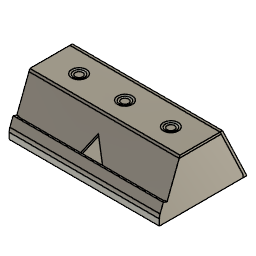
E-paper_v3 (Autodesk Fusion 360 design; units mm, degrees)
Autodesk Fusion 360 part; units mm, degrees
sketch "Sketch1" plane through (0, 0, 0) normal (1, 0, 0) x (0, 1, 0)
  line L0 (0, 0) -> (-90, 0)
  line L1 (-90, 0) -> (-54.1632, 93.358)
  line L2 (-90, 0) -> (10, 0) construction
  line L3 (0, -3.5) -> (-95.0925, -3.5)
  line L4 (-95.0925, -3.5) -> (-57.4307, 94.6123)
  line L5 (-58.8311, 95.1499) -> (-96.6992, -3.5)
  line L6 (-96.6992, -3.5) -> (-95.0925, -3.5)
  line L7 (-93.749, 0) -> (-95.3557, 0)
  line L8 (-96.6992, -3.5) -> (-100.1992, -3.5)
  line L9 (-100.1992, -3.5) -> (-62.3311, 95.1499)
  line L10 (-95.3557, 0) -> (-98.8557, 0)
  line L11 (-98.8557, 0) -> (-95.4512, 8.869)
  line L12 (-95.4512, 8.869) -> (-92.4007, 7.698)
  line L13 (-57.4307, 94.6123) -> (-54.1632, 93.358)
  line L14 (0, -3.5) -> (0, 0)
  line L15 (-92.4007, 7.698) -> (-91.0004, 7.1605)
  line L16 (-54.1632, 93.358) -> (0, 0)
  line L17 (-100.1992, -3.5) -> (0, -3.5) construction
  line L18 (0, -3.5) -> (0, -13.5)
  line L19 (0, -13.5) -> (-100.1992, -13.5)
  line L20 (-100.1992, -13.5) -> (-100.1992, -3.5)
  line L21 (0, -13.5) -> (0, -10)
  line L22 (0, -10) -> (-90, -10)
  line L23 (-90, -10) -> (-90, 0)
  dimension "d1" = 90
  dimension "d3" = 69
  dimension "d4" = 100
  dimension "d5" = -3.5
  dimension "d6" = 1.5
  dimension "d7" = 3.5
  dimension "d8" = 9.5
  dimension "d13" = 10
  dimension "d14" = 3.5
  constraint coincident L0.start L14.end
  constraint horizontal L0
  constraint horizontal L2
  constraint parallel L3 L6
  constraint coincident L4 L7.start
  constraint coincident L5 L7.end
  constraint parallel L6 L7
  constraint parallel L6 L8
  constraint parallel L5 L9
  constraint coincident L9 L10.end
  constraint parallel L7 L10
  constraint parallel L9 L11
  constraint coincident L5 L12.end
  constraint perpendicular L5 L12
  constraint perpendicular L1 L13
  constraint perpendicular L0 L14
  constraint coincident L4 L15.end
  constraint perpendicular L4 L15
  constraint horizontal L17
  constraint vertical L18
  constraint horizontal L19
  constraint vertical L20
  constraint perpendicular L19 L21
  constraint perpendicular L21 L22
  constraint perpendicular L17 L23
  measures "d1" distance of L0.start L0.end
  measures "d3" angle of L1 L2
  measures "d4" distance of L0.end L1.end
  measures "d6" distance of L4.end L5.start
  measures "d7" distance of L5.end L8.end
  measures "d8" distance of L10.end L11.end
  measures "d13" distance of L8.end L19.end
  measures "d14" distance of L18.end L21.end
extrude "Extrude1" add sketch "Sketch1" along normal blind 3 makes body 1
extrude "Extrude2" add sketch "Sketch1" against normal blind 174 contours L1 L3 L4 L13 L23 | L3 L6 L8 L18 L19 L20 L21 L22 L23 | L4 L5 L6 L7 | L5 L8 L9 L10 | L5 L9 L10 L11 L12 bodies 1
extrude "Extrude3" add sketch "Sketch1" against normal blind 3 from surface at -174 bodies 1
ref_plane "WorkPlane1" through (-87, -50.0996, 40.5562) normal (-1, 0, 0) x (0, 0, 1)
sketch "Sketch2" plane through (-87, 0, 0) normal (-1, 0, 0) x (0, -1, 0)
  arc A0 (90, -3.5) -> (95.35, 0) centre (90.3987, 1.7294) ccw
  line L0 (95.35, 0) -> (89.5, 0)
  line L1 (89.5, 0) -> (89.5, -3.5)
  line L2 (89.5, -3.5) -> (90, -3.5)
  constraint horizontal L0
  constraint perpendicular L0 L1
extrude "Extrude4" cut sketch "Sketch2" along normal mid plane 34 bodies 1
sketch "Sketch3" plane through (0, -81.709, 31.3652) normal (0, -0.93358, 0.358368) x (1, 0, 0)
  line L0 (0, -25.9267) -> (3, -25.9267)
  line L1 (3, -25.9267) -> (3, 67.7469)
  line L2 (3, 67.7469) -> (-177, 67.7469)
  line L3 (-177, 67.7469) -> (-177, -25.9267)
  line L4 (-177, -25.9267) -> (-174, -25.9267)
  line L5 (-174, -25.9267) -> (-174, -33.5966)
  line L6 (-174, -33.5966) -> (-104, -33.5966)
  line L7 (-104, -33.5966) -> (-70, -33.5966)
  line L8 (-70, -33.5966) -> (0, -33.5966)
  line L9 (0, -33.5966) -> (0, -25.9267)
  line L10 (-104, -33.5966) -> (-87.5, -3)
  line L11 (-87.5, -3) -> (-70, -33.5966)
  line L12 (-104, -33.5966) -> (-70, -33.5966)
  constraint coincident L6.end L7.start
  constraint coincident L7.end L8.start
extrude "Extrude5" cut sketch "Sketch3" against normal blind 5 contours L7 L10 L11 L12 bodies 1
sketch "Sketch4" plane through (0, -90, 0) normal (0, 1, 0) x (-1, 0, 0)
  line L0 (104, 0) -> (104, -3.5)
  line L1 (104, -3.5) -> (70, -3.5)
  line L2 (70, -3.5) -> (70, 0)
  line L3 (70, 0) -> (0, 0)
  line L4 (0, 0) -> (0, -10)
  line L5 (0, -10) -> (174, -10)
  line L6 (174, -10) -> (174, 0)
  line L7 (174, 0) -> (104, 0)
  line L8 (12.6874, -4.866) -> (9.8668, -2.0298)
  line L9 (9.8668, -2.0298) -> (7.0306, -4.8504)
  line L10 (7.0306, -4.8504) -> (9.8511, -7.6866)
  line L11 (9.8511, -7.6866) -> (12.6874, -4.866)
  line L12 (40.6511, -7.6866) -> (43.4874, -4.866)
  line L13 (37.8306, -4.8504) -> (40.6511, -7.6866)
  line L14 (40.6668, -2.0298) -> (37.8306, -4.8504)
  line L15 (43.4874, -4.866) -> (40.6668, -2.0298)
  line L16 (71.4511, -7.6866) -> (74.2874, -4.866)
  line L17 (68.6306, -4.8504) -> (71.4511, -7.6866)
  line L18 (71.4668, -2.0298) -> (68.6306, -4.8504)
  line L19 (74.2874, -4.866) -> (71.4668, -2.0298)
  line L20 (102.2511, -7.6866) -> (105.0874, -4.866)
  line L21 (99.4306, -4.8504) -> (102.2511, -7.6866)
  line L22 (102.2668, -2.0298) -> (99.4306, -4.8504)
  line L23 (105.0874, -4.866) -> (102.2668, -2.0298)
  line L24 (133.0511, -7.6866) -> (135.8874, -4.866)
  line L25 (130.2306, -4.8504) -> (133.0511, -7.6866)
  line L26 (133.0668, -2.0298) -> (130.2306, -4.8504)
  line L27 (135.8874, -4.866) -> (133.0668, -2.0298)
  line L28 (163.8511, -7.6866) -> (166.6874, -4.866)
  line L29 (161.0306, -4.8504) -> (163.8511, -7.6866)
  line L30 (163.8668, -2.0298) -> (161.0306, -4.8504)
  line L31 (166.6874, -4.866) -> (163.8668, -2.0298)
  point P0 (9.859, -4.8582)
  point P1 (40.659, -4.8582)
  point P2 (71.459, -4.8582)
  point P3 (102.259, -4.8582)
  point P4 (133.059, -4.8582)
  point P5 (163.859, -4.8582)
  dimension "d22" = 2
  dimension "d25" = 154
  dimension "d26" = 0
  measures "d22" distance of P0 L11
sketch "Sketch5" plane through (0, -90, 0) normal (0, 1, 0) x (-1, 0, 0)
extrude "Extrude6" cut sketch "Sketch4" against normal blind 8.8 contours L1 L20 L21 L22 L23 | L1 L22 L23 | L1 L2 L16 L17 L18 L19 | L1 L2 L18 L19 | L8 L9 L10 L11 | L12 L13 L14 L15 | L24 L25 L26 L27 | L28 L29 L30 L31 bodies 1
sketch "Sketch6" plane through (3, 0, 0) normal (1, 0, 0) x (0, 1, 0)
  line L0 (-100.1992, -13.5) -> (0, -13.5)
  line L1 (0, -13.5) -> (0, 0)
  line L2 (0, 0) -> (-54.1632, 93.358)
  line L3 (-54.1632, 93.358) -> (-57.4307, 94.6123)
  line L4 (-57.4307, 94.6123) -> (-91.0004, 7.1605)
  line L5 (-91.0004, 7.1605) -> (-95.4512, 8.869)
  line L6 (-95.4512, 8.869) -> (-100.1992, -3.5)
  line L7 (-100.1992, -3.5) -> (-100.1992, -13.5)
  line L8 (-100, 45) -> (0, 45)
  line L9 (0, 45) -> (0, 100)
  line L10 (0, 100) -> (-100, 100)
  line L11 (-100, 100) -> (-100, 45)
  constraint horizontal L8
  constraint vertical L9
  constraint horizontal L10
  constraint vertical L11
extrude "Extrude7" cut sketch "Sketch6" against normal blind 200 contours L2 L3 L4 L8 bodies 1
fillet "Fillet1" radius 13 1 edges at (-87, -100.1992, -3.5) on bodies 1
sketch "Sketch7" plane through (-177, 0, 0) normal (-1, 0, 0) x (0, -1, 0)
  arc A0 (100.1992, -5.9094) -> (99.3358, -1.2506) centre (87.1992, -5.9094) ccw
  line L0 (99.3358, -1.2506) -> (95.4512, 8.869)
  line L1 (95.4512, 8.869) -> (91.0004, 7.1605)
  line L2 (91.0004, 7.1605) -> (76.4751, 45)
  line L3 (76.4751, 45) -> (26.1075, 45)
  line L4 (26.1075, 45) -> (0, 0)
  line L5 (0, 0) -> (0, -13.5)
  line L6 (0, -13.5) -> (100.1992, -13.5)
  line L7 (100.1992, -13.5) -> (100.1992, -5.9094)
  line L8 (0, -10) -> (26.1075, 45)
  line L9 (-5, 45) -> (26.1075, 45)
  line L10 (-5, 45) -> (0, -10)
  constraint coincident L5 L8.start
  constraint coincident L3.end L4.start
  constraint parallel L3 L9
extrude "Extrude8" cut sketch "Sketch7" against normal blind 225 contours L4 L5 L8 bodies 1
sketch "Sketch8" plane through (0, 0, -13.5) normal (0, 0, -1) x (1, 0, 0)
  line L0 (-177, 0) -> (3, 0)
  line L1 (3, 0) -> (3, 100.1992)
  line L2 (3, 100.1992) -> (-177, 100.1992)
  line L3 (-177, 100.1992) -> (-177, 0)
  line L4 (-25, 60) -> (-28.8404, 50)
  line L5 (-28.8404, 50) -> (-30.266, 50)
  line L6 (-30.266, 50) -> (-34.3588, 60)
  line L7 (-34.3588, 60) -> (-32.8513, 60)
  line L8 (-32.8513, 60) -> (-31.6849, 56.9714)
  line L9 (-31.6849, 56.9714) -> (-27.5034, 56.9714)
  line L10 (-27.5034, 56.9714) -> (-26.4052, 60)
  line L11 (-26.4052, 60) -> (-25, 60)
  line L12 (-27.8854, 55.8936) -> (-31.2756, 55.8936)
  line L13 (-31.2756, 55.8936) -> (-30.2319, 53.1241)
  spline S0 degree 2 poles (-30.2319, 53.1241) (-29.7544, 51.8622) (-29.5225, 51.0505) knots 0 0 0 1 1 1
  spline S1 degree 2 poles (-29.5225, 51.0505) (-29.3315, 52.0123) (-28.9836, 52.9604) knots 0 0 0 1 1 1
  line L14 (-28.9836, 52.9604) -> (-27.8854, 55.8936)
  line L15 (-35.2319, 60) -> (-35.2319, 50)
  line L16 (-35.2319, 50) -> (-36.4598, 50)
  line L17 (-36.4598, 50) -> (-36.4598, 60)
  line L18 (-36.4598, 60) -> (-35.2319, 60)
  line L19 (-43.322, 57.6671) -> (-44.5907, 57.824)
  spline S2 degree 2 poles (-44.5907, 57.824) (-44.2906, 58.9359) (-43.4789, 59.5498) knots 0 0 0 1 1 1
  spline S3 degree 2 poles (-43.4789, 59.5498) (-42.6671, 60.1637) (-41.4052, 60.1637) knots 0 0 0 1 1 1
  spline S4 degree 2 poles (-41.4052, 60.1637) (-39.8158, 60.1637) (-38.8847, 59.1849) knots 0 0 0 1 1 1
  spline S5 degree 2 poles (-38.8847, 59.1849) (-37.9536, 58.206) (-37.9536, 56.4393) knots 0 0 0 1 1 1
  spline S6 degree 2 poles (-37.9536, 56.4393) (-37.9536, 54.6112) (-38.895, 53.6016) knots 0 0 0 1 1 1
  spline S7 degree 2 poles (-38.895, 53.6016) (-39.8363, 52.5921) (-41.337, 52.5921) knots 0 0 0 1 1 1
  spline S8 degree 2 poles (-41.337, 52.5921) (-42.7899, 52.5921) (-43.7108, 53.5812) knots 0 0 0 1 1 1
  spline S9 degree 2 poles (-43.7108, 53.5812) (-44.6317, 54.5703) (-44.6317, 56.3643) knots 0 0 0 1 1 1
  spline S10 degree 2 poles (-44.6317, 56.3643) (-44.6317, 56.4734) (-44.6248, 56.6917) knots 0 0 0 1 1 1
  line L20 (-44.6248, 56.6917) -> (-39.2224, 56.6917)
  spline S11 degree 2 poles (-39.2224, 56.6917) (-39.2906, 57.8854) (-39.8977, 58.5198) knots 0 0 0 1 1 1
  spline S12 degree 2 poles (-39.8977, 58.5198) (-40.5048, 59.1542) (-41.412, 59.1542) knots 0 0 0 1 1 1
  spline S13 degree 2 poles (-41.412, 59.1542) (-42.0873, 59.1542) (-42.5648, 58.7995) knots 0 0 0 1 1 1
  spline S14 degree 2 poles (-42.5648, 58.7995) (-43.0423, 58.4447) (-43.322, 57.6671) knots 0 0 0 1 1 1
  line L21 (-39.2906, 55.6821) -> (-43.3356, 55.6821)
  spline S15 degree 2 poles (-43.3356, 55.6821) (-43.2538, 54.7681) (-42.8718, 54.3111) knots 0 0 0 1 1 1
  spline S16 degree 2 poles (-42.8718, 54.3111) (-42.2851, 53.6016) (-41.3506, 53.6016) knots 0 0 0 1 1 1
  spline S17 degree 2 poles (-41.3506, 53.6016) (-40.5048, 53.6016) (-39.9284, 54.1678) knots 0 0 0 1 1 1
  spline S18 degree 2 poles (-39.9284, 54.1678) (-39.352, 54.734) (-39.2906, 55.6821) knots 0 0 0 1 1 1
  line L22 (-54.8499, 56.0778) -> (-54.8499, 54.9045)
  line L23 (-54.8499, 54.9045) -> (-59.0859, 54.8977)
  line L24 (-59.0859, 54.8977) -> (-59.0859, 58.6085)
  spline S19 degree 2 poles (-59.0859, 58.6085) (-58.1105, 59.3861) (-57.0737, 59.7783) knots 0 0 0 1 1 1
  spline S20 degree 2 poles (-57.0737, 59.7783) (-56.0368, 60.1705) (-54.9454, 60.1705) knots 0 0 0 1 1 1
  spline S21 degree 2 poles (-54.9454, 60.1705) (-53.472, 60.1705) (-52.2681, 59.5396) knots 0 0 0 1 1 1
  spline S22 degree 2 poles (-52.2681, 59.5396) (-51.0641, 58.9086) (-50.4502, 57.7149) knots 0 0 0 1 1 1
  spline S23 degree 2 poles (-50.4502, 57.7149) (-49.8363, 56.5211) (-49.8363, 55.0478) knots 0 0 0 1 1 1
  spline S24 degree 2 poles (-49.8363, 55.0478) (-49.8363, 53.588) (-50.4468, 52.3226) knots 0 0 0 1 1 1
  spline S25 degree 2 poles (-50.4468, 52.3226) (-51.0573, 51.0573) (-52.2033, 50.4434) knots 0 0 0 1 1 1
  spline S26 degree 2 poles (-52.2033, 50.4434) (-53.3493, 49.8295) (-54.8431, 49.8295) knots 0 0 0 1 1 1
  spline S27 degree 2 poles (-54.8431, 49.8295) (-55.9277, 49.8295) (-56.8042, 50.1808) knots 0 0 0 1 1 1
  spline S28 degree 2 poles (-56.8042, 50.1808) (-57.6808, 50.5321) (-58.1787, 51.1596) knots 0 0 0 1 1 1
  spline S29 degree 2 poles (-58.1787, 51.1596) (-58.6767, 51.7872) (-58.9359, 52.7967) knots 0 0 0 1 1 1
  line L25 (-58.9359, 52.7967) -> (-57.7422, 53.1241)
  spline S30 degree 2 poles (-57.7422, 53.1241) (-57.5171, 52.3602) (-57.1828, 51.9236) knots 0 0 0 1 1 1
  spline S31 degree 2 poles (-57.1828, 51.9236) (-56.8486, 51.487) (-56.2278, 51.2244) knots 0 0 0 1 1 1
  spline S32 degree 2 poles (-56.2278, 51.2244) (-55.6071, 50.9618) (-54.8499, 50.9618) knots 0 0 0 1 1 1
  spline S33 degree 2 poles (-54.8499, 50.9618) (-53.9427, 50.9618) (-53.281, 51.2381) knots 0 0 0 1 1 1
  spline S34 degree 2 poles (-53.281, 51.2381) (-52.6194, 51.5143) (-52.2135, 51.9645) knots 0 0 0 1 1 1
  spline S35 degree 2 poles (-52.2135, 51.9645) (-51.8076, 52.4147) (-51.5825, 52.9536) knots 0 0 0 1 1 1
  spline S36 degree 2 poles (-51.5825, 52.9536) (-51.2005, 53.8813) (-51.2005, 54.9659) knots 0 0 0 1 1 1
  spline S37 degree 2 poles (-51.2005, 54.9659) (-51.2005, 56.3029) (-51.661, 57.2033) knots 0 0 0 1 1 1
  spline S38 degree 2 poles (-51.661, 57.2033) (-52.1214, 58.1037) (-53.0014, 58.5402) knots 0 0 0 1 1 1
  spline S39 degree 2 poles (-53.0014, 58.5402) (-53.8813, 58.9768) (-54.8704, 58.9768) knots 0 0 0 1 1 1
  spline S40 degree 2 poles (-54.8704, 58.9768) (-55.7299, 58.9768) (-56.5484, 58.646) knots 0 0 0 1 1 1
  spline S41 degree 2 poles (-56.5484, 58.646) (-57.367, 58.3151) (-57.7899, 57.94) knots 0 0 0 1 1 1
  line L26 (-57.7899, 57.94) -> (-57.7899, 56.0778)
  line L27 (-57.7899, 56.0778) -> (-54.8499, 56.0778)
  spline S42 degree 2 poles (-32.94, 74.4952) (-32.4966, 75.0068) (-31.9475, 75.3172) knots 0 0 0 1 1 1
  spline S43 degree 2 poles (-31.9475, 75.3172) (-31.3984, 75.6276) (-30.8458, 75.6276) knots 0 0 0 1 1 1
  spline S44 degree 2 poles (-30.8458, 75.6276) (-30.2387, 75.6276) (-29.6658, 75.2729) knots 0 0 0 1 1 1
  spline S45 degree 2 poles (-29.6658, 75.2729) (-29.0928, 74.9181) (-28.7347, 74.1814) knots 0 0 0 1 1 1
  spline S46 degree 2 poles (-28.7347, 74.1814) (-28.3765, 73.4447) (-28.3765, 72.5648) knots 0 0 0 1 1 1
  spline S47 degree 2 poles (-28.3765, 72.5648) (-28.3765, 71.4802) (-28.9325, 70.3922) knots 0 0 0 1 1 1
  spline S48 degree 2 poles (-28.9325, 70.3922) (-29.4884, 69.3042) (-30.3138, 68.7585) knots 0 0 0 1 1 1
  spline S49 degree 2 poles (-30.3138, 68.7585) (-31.1392, 68.2128) (-31.9168, 68.2128) knots 0 0 0 1 1 1
  spline S50 degree 2 poles (-31.9168, 68.2128) (-32.5102, 68.2128) (-33.0491, 68.5232) knots 0 0 0 1 1 1
  spline S51 degree 2 poles (-33.0491, 68.5232) (-33.588, 68.8336) (-33.9768, 69.4679) knots 0 0 0 1 1 1
  line L28 (-33.9768, 69.4679) -> (-34.2087, 68.4106)
  line L29 (-34.2087, 68.4106) -> (-35.4297, 68.4106)
  line L30 (-35.4297, 68.4106) -> (-34.4475, 72.9877)
  spline S52 degree 2 poles (-34.4475, 72.9877) (-34.2428, 73.9427) (-34.2428, 74.045) knots 0 0 0 1 1 1
  spline S53 degree 2 poles (-34.2428, 74.045) (-34.2428, 74.2292) (-34.3827, 74.3622) knots 0 0 0 1 1 1
  spline S54 degree 2 poles (-34.3827, 74.3622) (-34.5225, 74.4952) (-34.7203, 74.4952) knots 0 0 0 1 1 1
  spline S55 degree 2 poles (-34.7203, 74.4952) (-35.0819, 74.4952) (-35.6685, 74.0791) knots 0 0 0 1 1 1
  spline S56 degree 2 poles (-35.6685, 74.0791) (-36.4461, 73.5334) (-36.8997, 72.616) knots 0 0 0 1 1 1
  spline S57 degree 2 poles (-36.8997, 72.616) (-37.3533, 71.6985) (-37.3533, 70.7231) knots 0 0 0 1 1 1
  spline S58 degree 2 poles (-37.3533, 70.7231) (-37.3533, 69.5839) (-36.7701, 68.5948) knots 0 0 0 1 1 1
  spline S59 degree 2 poles (-36.7701, 68.5948) (-36.1869, 67.6057) (-35.0307, 67.0123) knots 0 0 0 1 1 1
  spline S60 degree 2 poles (-35.0307, 67.0123) (-33.8745, 66.4188) (-32.4761, 66.4188) knots 0 0 0 1 1 1
  spline S61 degree 2 poles (-32.4761, 66.4188) (-30.8799, 66.4188) (-29.56, 67.1658) knots 0 0 0 1 1 1
  spline S62 degree 2 poles (-29.56, 67.1658) (-28.2401, 67.9127) (-27.5136, 69.3076) knots 0 0 0 1 1 1
  spline S63 degree 2 poles (-27.5136, 69.3076) (-26.7872, 70.7026) (-26.7872, 72.2988) knots 0 0 0 1 1 1
  spline S64 degree 2 poles (-26.7872, 72.2988) (-26.7872, 73.97) (-27.5136, 75.1774) knots 0 0 0 1 1 1
  spline S65 degree 2 poles (-27.5136, 75.1774) (-28.2401, 76.3847) (-29.6146, 76.9611) knots 0 0 0 1 1 1
  spline S66 degree 2 poles (-29.6146, 76.9611) (-30.9891, 77.5375) (-32.6603, 77.5375) knots 0 0 0 1 1 1
  spline S67 degree 2 poles (-32.6603, 77.5375) (-34.4475, 77.5375) (-35.6548, 76.9372) knots 0 0 0 1 1 1
  spline S68 degree 2 poles (-35.6548, 76.9372) (-36.8622, 76.337) (-37.4625, 75.4775) knots 0 0 0 1 1 1
  line L31 (-37.4625, 75.4775) -> (-38.6971, 75.4775)
  spline S69 degree 2 poles (-38.6971, 75.4775) (-38.3493, 76.1937) (-37.5034, 76.9372) knots 0 0 0 1 1 1
  spline S70 degree 2 poles (-37.5034, 76.9372) (-36.6576, 77.6808) (-35.4911, 78.1139) knots 0 0 0 1 1 1
  spline S71 degree 2 poles (-35.4911, 78.1139) (-34.3247, 78.5471) (-32.6808, 78.5471) knots 0 0 0 1 1 1
  spline S72 degree 2 poles (-32.6808, 78.5471) (-31.1664, 78.5471) (-29.8874, 78.1583) knots 0 0 0 1 1 1
  spline S73 degree 2 poles (-29.8874, 78.1583) (-28.6085, 77.7694) (-27.708, 76.9884) knots 0 0 0 1 1 1
  spline S74 degree 2 poles (-27.708, 76.9884) (-26.8076, 76.2074) (-26.3506, 75.191) knots 0 0 0 1 1 1
  spline S75 degree 2 poles (-26.3506, 75.191) (-25.7776, 73.9018) (-25.7776, 72.4079) knots 0 0 0 1 1 1
  spline S76 degree 2 poles (-25.7776, 72.4079) (-25.7776, 70.7435) (-26.4598, 69.236) knots 0 0 0 1 1 1
  spline S77 degree 2 poles (-26.4598, 69.236) (-27.292, 67.3874) (-28.8233, 66.4052) knots 0 0 0 1 1 1
  spline S78 degree 2 poles (-28.8233, 66.4052) (-30.3547, 65.4229) (-32.5375, 65.4229) knots 0 0 0 1 1 1
  spline S79 degree 2 poles (-32.5375, 65.4229) (-34.2292, 65.4229) (-35.5764, 66.1153) knots 0 0 0 1 1 1
  spline S80 degree 2 poles (-35.5764, 66.1153) (-36.9236, 66.8076) (-37.7012, 68.1787) knots 0 0 0 1 1 1
  spline S81 degree 2 poles (-37.7012, 68.1787) (-38.3629, 69.3588) (-38.3629, 70.7435) knots 0 0 0 1 1 1
  spline S82 degree 2 poles (-38.3629, 70.7435) (-38.3629, 72.7217) (-36.9714, 74.2565) knots 0 0 0 1 1 1
  spline S83 degree 2 poles (-36.9714, 74.2565) (-35.7299, 75.6344) (-34.2565, 75.6344) knots 0 0 0 1 1 1
  spline S84 degree 2 poles (-34.2565, 75.6344) (-33.7858, 75.6344) (-33.4959, 75.4911) knots 0 0 0 1 1 1
  spline S85 degree 2 poles (-33.4959, 75.4911) (-33.206, 75.3479) (-33.0696, 75.0819) knots 0 0 0 1 1 1
  spline S86 degree 2 poles (-33.0696, 75.0819) (-32.9809, 74.9113) (-32.94, 74.4952) knots 0 0 0 1 1 1
  spline S87 degree 2 poles (-29.6385, 72.6467) (-29.6385, 73.5812) (-30.0819, 74.0996) knots 0 0 0 1 1 1
  spline S88 degree 2 poles (-30.0819, 74.0996) (-30.5252, 74.618) (-31.0982, 74.618) knots 0 0 0 1 1 1
  spline S89 degree 2 poles (-31.0982, 74.618) (-31.4802, 74.618) (-31.9031, 74.3895) knots 0 0 0 1 1 1
  spline S90 degree 2 poles (-31.9031, 74.3895) (-32.3261, 74.161) (-32.7115, 73.7108) knots 0 0 0 1 1 1
  spline S91 degree 2 poles (-32.7115, 73.7108) (-33.0969, 73.2606) (-33.3424, 72.5682) knots 0 0 0 1 1 1
  spline S92 degree 2 poles (-33.3424, 72.5682) (-33.588, 71.8759) (-33.588, 71.1801) knots 0 0 0 1 1 1
  spline S93 degree 2 poles (-33.588, 71.1801) (-33.588, 70.2524) (-33.1276, 69.7408) knots 0 0 0 1 1 1
  spline S94 degree 2 poles (-33.1276, 69.7408) (-32.6671, 69.2292) (-32.0055, 69.2292) knots 0 0 0 1 1 1
  spline S95 degree 2 poles (-32.0055, 69.2292) (-31.5689, 69.2292) (-31.1835, 69.4509) knots 0 0 0 1 1 1
  spline S96 degree 2 poles (-31.1835, 69.4509) (-30.7981, 69.6726) (-30.4366, 70.1637) knots 0 0 0 1 1 1
  spline S97 degree 2 poles (-30.4366, 70.1637) (-30.075, 70.6548) (-29.8568, 71.3574) knots 0 0 0 1 1 1
  spline S98 degree 2 poles (-29.8568, 71.3574) (-29.6385, 72.06) (-29.6385, 72.6467) knots 0 0 0 1 1 1
  line L32 (-46.2347, 74.427) -> (-46.2347, 75.6071)
  line L33 (-46.2347, 75.6071) -> (-39.6248, 75.6071)
  spline S99 degree 2 poles (-39.6248, 75.6071) (-39.6112, 75.1637) (-39.7681, 74.7544) knots 0 0 0 1 1 1
  spline S100 degree 2 poles (-39.7681, 74.7544) (-40.0205, 74.0791) (-40.5764, 73.4243) knots 0 0 0 1 1 1
  spline S101 degree 2 poles (-40.5764, 73.4243) (-41.1323, 72.7694) (-42.1828, 71.91) knots 0 0 0 1 1 1
  spline S102 degree 2 poles (-42.1828, 71.91) (-43.8131, 70.573) (-44.3861, 69.792) knots 0 0 0 1 1 1
  spline S103 degree 2 poles (-44.3861, 69.792) (-44.9591, 69.0109) (-44.9591, 68.3151) knots 0 0 0 1 1 1
  spline S104 degree 2 poles (-44.9591, 68.3151) (-44.9591, 67.5853) (-44.4372, 67.0839) knots 0 0 0 1 1 1
  spline S105 degree 2 poles (-44.4372, 67.0839) (-43.9154, 66.5825) (-43.0764, 66.5825) knots 0 0 0 1 1 1
  spline S106 degree 2 poles (-43.0764, 66.5825) (-42.1896, 66.5825) (-41.6576, 67.1146) knots 0 0 0 1 1 1
  spline S107 degree 2 poles (-41.6576, 67.1146) (-41.1255, 67.6467) (-41.1187, 68.588) knots 0 0 0 1 1 1
  line L34 (-41.1187, 68.588) -> (-39.8568, 68.4584)
  spline S108 degree 2 poles (-39.8568, 68.4584) (-39.9864, 67.0464) (-40.8322, 66.3063) knots 0 0 0 1 1 1
  spline S109 degree 2 poles (-40.8322, 66.3063) (-41.678, 65.5662) (-43.1037, 65.5662) knots 0 0 0 1 1 1
  spline S110 degree 2 poles (-43.1037, 65.5662) (-44.543, 65.5662) (-45.382, 66.3643) knots 0 0 0 1 1 1
  spline S111 degree 2 poles (-45.382, 66.3643) (-46.221, 67.1623) (-46.221, 68.3424) knots 0 0 0 1 1 1
  spline S112 degree 2 poles (-46.221, 68.3424) (-46.221, 68.9427) (-45.9754, 69.5225) knots 0 0 0 1 1 1
  spline S113 degree 2 poles (-45.9754, 69.5225) (-45.7299, 70.1023) (-45.1603, 70.7435) knots 0 0 0 1 1 1
  spline S114 degree 2 poles (-45.1603, 70.7435) (-44.5907, 71.3847) (-43.2674, 72.5034) knots 0 0 0 1 1 1
  spline S115 degree 2 poles (-43.2674, 72.5034) (-42.1623, 73.4311) (-41.8486, 73.7619) knots 0 0 0 1 1 1
  spline S116 degree 2 poles (-41.8486, 73.7619) (-41.5348, 74.0928) (-41.3301, 74.427) knots 0 0 0 1 1 1
  line L35 (-41.3301, 74.427) -> (-46.2347, 74.427)
  spline S117 degree 2 poles (-47.5512, 70.6753) (-47.5512, 68.9018) (-47.9161, 67.8206) knots 0 0 0 1 1 1
  spline S118 degree 2 poles (-47.9161, 67.8206) (-48.281, 66.7394) (-49.0007, 66.1528) knots 0 0 0 1 1 1
  spline S119 degree 2 poles (-49.0007, 66.1528) (-49.7203, 65.5662) (-50.8117, 65.5662) knots 0 0 0 1 1 1
  spline S120 degree 2 poles (-50.8117, 65.5662) (-51.6166, 65.5662) (-52.2237, 65.8902) knots 0 0 0 1 1 1
  spline S121 degree 2 poles (-52.2237, 65.8902) (-52.8308, 66.2142) (-53.2265, 66.8247) knots 0 0 0 1 1 1
  spline S122 degree 2 poles (-53.2265, 66.8247) (-53.6221, 67.4352) (-53.8472, 68.3117) knots 0 0 0 1 1 1
  spline S123 degree 2 poles (-53.8472, 68.3117) (-54.0723, 69.1883) (-54.0723, 70.6753) knots 0 0 0 1 1 1
  spline S124 degree 2 poles (-54.0723, 70.6753) (-54.0723, 72.4352) (-53.7108, 73.5164) knots 0 0 0 1 1 1
  spline S125 degree 2 poles (-53.7108, 73.5164) (-53.3493, 74.5975) (-52.6296, 75.1876) knots 0 0 0 1 1 1
  spline S126 degree 2 poles (-52.6296, 75.1876) (-51.91, 75.7776) (-50.8117, 75.7776) knots 0 0 0 1 1 1
  spline S127 degree 2 poles (-50.8117, 75.7776) (-49.3656, 75.7776) (-48.5402, 74.7408) knots 0 0 0 1 1 1
  spline S128 degree 2 poles (-48.5402, 74.7408) (-47.5512, 73.4925) (-47.5512, 70.6753) knots 0 0 0 1 1 1
  spline S129 degree 2 poles (-48.8131, 70.6753) (-48.8131, 73.1378) (-49.3895, 73.9529) knots 0 0 0 1 1 1
  spline S130 degree 2 poles (-49.3895, 73.9529) (-49.9659, 74.7681) (-50.8117, 74.7681) knots 0 0 0 1 1 1
  spline S131 degree 2 poles (-50.8117, 74.7681) (-51.6576, 74.7681) (-52.234, 73.9495) knots 0 0 0 1 1 1
  spline S132 degree 2 poles (-52.234, 73.9495) (-52.8104, 73.131) (-52.8104, 70.6753) knots 0 0 0 1 1 1
  spline S133 degree 2 poles (-52.8104, 70.6753) (-52.8104, 68.206) (-52.234, 67.3943) knots 0 0 0 1 1 1
  spline S134 degree 2 poles (-52.234, 67.3943) (-51.6576, 66.5825) (-50.7981, 66.5825) knots 0 0 0 1 1 1
  spline S135 degree 2 poles (-50.7981, 66.5825) (-49.9523, 66.5825) (-49.4475, 67.2988) knots 0 0 0 1 1 1
  spline S136 degree 2 poles (-49.4475, 67.2988) (-48.8131, 68.2128) (-48.8131, 70.6753) knots 0 0 0 1 1 1
  line L36 (-61.7735, 74.427) -> (-61.7735, 75.6071)
  line L37 (-61.7735, 75.6071) -> (-55.1637, 75.6071)
  spline S137 degree 2 poles (-55.1637, 75.6071) (-55.1501, 75.1637) (-55.307, 74.7544) knots 0 0 0 1 1 1
  spline S138 degree 2 poles (-55.307, 74.7544) (-55.5593, 74.0791) (-56.1153, 73.4243) knots 0 0 0 1 1 1
  spline S139 degree 2 poles (-56.1153, 73.4243) (-56.6712, 72.7694) (-57.7217, 71.91) knots 0 0 0 1 1 1
  spline S140 degree 2 poles (-57.7217, 71.91) (-59.352, 70.573) (-59.925, 69.792) knots 0 0 0 1 1 1
  spline S141 degree 2 poles (-59.925, 69.792) (-60.498, 69.0109) (-60.498, 68.3151) knots 0 0 0 1 1 1
  spline S142 degree 2 poles (-60.498, 68.3151) (-60.498, 67.5853) (-59.9761, 67.0839) knots 0 0 0 1 1 1
  spline S143 degree 2 poles (-59.9761, 67.0839) (-59.4543, 66.5825) (-58.6153, 66.5825) knots 0 0 0 1 1 1
  spline S144 degree 2 poles (-58.6153, 66.5825) (-57.7285, 66.5825) (-57.1965, 67.1146) knots 0 0 0 1 1 1
  spline S145 degree 2 poles (-57.1965, 67.1146) (-56.6644, 67.6467) (-56.6576, 68.588) knots 0 0 0 1 1 1
  line L38 (-56.6576, 68.588) -> (-55.3956, 68.4584)
  spline S146 degree 2 poles (-55.3956, 68.4584) (-55.5252, 67.0464) (-56.3711, 66.3063) knots 0 0 0 1 1 1
  spline S147 degree 2 poles (-56.3711, 66.3063) (-57.2169, 65.5662) (-58.6426, 65.5662) knots 0 0 0 1 1 1
  spline S148 degree 2 poles (-58.6426, 65.5662) (-60.0819, 65.5662) (-60.9209, 66.3643) knots 0 0 0 1 1 1
  spline S149 degree 2 poles (-60.9209, 66.3643) (-61.7599, 67.1623) (-61.7599, 68.3424) knots 0 0 0 1 1 1
  spline S150 degree 2 poles (-61.7599, 68.3424) (-61.7599, 68.9427) (-61.5143, 69.5225) knots 0 0 0 1 1 1
  spline S151 degree 2 poles (-61.5143, 69.5225) (-61.2688, 70.1023) (-60.6992, 70.7435) knots 0 0 0 1 1 1
  spline S152 degree 2 poles (-60.6992, 70.7435) (-60.1296, 71.3847) (-58.8063, 72.5034) knots 0 0 0 1 1 1
  spline S153 degree 2 poles (-58.8063, 72.5034) (-57.7012, 73.4311) (-57.3874, 73.7619) knots 0 0 0 1 1 1
  spline S154 degree 2 poles (-57.3874, 73.7619) (-57.0737, 74.0928) (-56.869, 74.427) knots 0 0 0 1 1 1
  line L39 (-56.869, 74.427) -> (-61.7735, 74.427)
  line L40 (-63.09, 72.9877) -> (-64.3793, 72.8786)
  spline S155 degree 2 poles (-64.3793, 72.8786) (-64.5225, 73.8199) (-65.0443, 74.294) knots 0 0 0 1 1 1
  spline S156 degree 2 poles (-65.0443, 74.294) (-65.5662, 74.7681) (-66.3029, 74.7681) knots 0 0 0 1 1 1
  spline S157 degree 2 poles (-66.3029, 74.7681) (-67.1896, 74.7681) (-67.8035, 74.0996) knots 0 0 0 1 1 1
  spline S158 degree 2 poles (-67.8035, 74.0996) (-68.4175, 73.4311) (-68.4175, 72.3261) knots 0 0 0 1 1 1
  spline S159 degree 2 poles (-68.4175, 72.3261) (-68.4175, 71.2756) (-67.8274, 70.6685) knots 0 0 0 1 1 1
  spline S160 degree 2 poles (-67.8274, 70.6685) (-67.2374, 70.0614) (-66.2824, 70.0614) knots 0 0 0 1 1 1
  spline S161 degree 2 poles (-66.2824, 70.0614) (-65.689, 70.0614) (-65.2115, 70.3308) knots 0 0 0 1 1 1
  spline S162 degree 2 poles (-65.2115, 70.3308) (-64.734, 70.6003) (-64.4611, 71.03) knots 0 0 0 1 1 1
  line L41 (-64.4611, 71.03) -> (-63.3083, 70.8799)
  line L42 (-63.3083, 70.8799) -> (-64.2769, 65.7435)
  line L43 (-64.2769, 65.7435) -> (-69.2497, 65.7435)
  line L44 (-69.2497, 65.7435) -> (-69.2497, 66.9168)
  line L45 (-69.2497, 66.9168) -> (-65.2592, 66.9168)
  line L46 (-65.2592, 66.9168) -> (-64.7203, 69.6044)
  spline S163 degree 2 poles (-64.7203, 69.6044) (-65.6207, 68.9768) (-66.6098, 68.9768) knots 0 0 0 1 1 1
  spline S164 degree 2 poles (-66.6098, 68.9768) (-67.9195, 68.9768) (-68.8199, 69.884) knots 0 0 0 1 1 1
  spline S165 degree 2 poles (-68.8199, 69.884) (-69.7203, 70.7913) (-69.7203, 72.2169) knots 0 0 0 1 1 1
  spline S166 degree 2 poles (-69.7203, 72.2169) (-69.7203, 73.5744) (-68.9291, 74.5634) knots 0 0 0 1 1 1
  spline S167 degree 2 poles (-68.9291, 74.5634) (-67.9673, 75.7776) (-66.3029, 75.7776) knots 0 0 0 1 1 1
  spline S168 degree 2 poles (-66.3029, 75.7776) (-64.9386, 75.7776) (-64.0757, 75.0136) knots 0 0 0 1 1 1
  spline S169 degree 2 poles (-64.0757, 75.0136) (-63.2128, 74.2497) (-63.09, 72.9877) knots 0 0 0 1 1 1
extrude "Extrude9" cut sketch "Sketch8" against normal blind 0.5 contours L4 L5 L6 L7 L8 L9 L10 L11 | L15 L16 L17 L18 | L19 S2 S3 S4 S5 S6 S7 S8 S9 S10 L20 S11 S12 S13 S14 | L22 L23 L24 S19 S20 S21 S22 S23 S24 S25 S26 S27 S28 S29 L25 S30 S31 S32 S33 S34 S35 S36 S37 S38 S39 S40 S41 L26 L27 | S42 S43 S44 S45 S46 S47 S48 S49 S50 S51 L28 L29 L30 S52 S53 S54 S55 S56 S57 S58 S59 S60 S61 S62 S63 S64 S65 S66 S67 S68 L31 S69 S70 S71 S72 S73 S74 S75 S76 S77 S78 S79 S80 S81 S82 S83 S84 S85 S86 | L32 L33 S99 S100 S101 S102 S103 S104 S105 S106 S107 L34 S108 S109 S110 S111 S112 S113 S114 S115 S116 L35 | S117 S118 S119 S120 S121 S122 S123 S124 S125 S126 S127 S128 | L36 L37 S137 S138 S139 S140 S141 S142 S143 S144 S145 L38 S146 S147 S148 S149 S150 S151 S152 S153 S154 L39 | L40 S155 S156 S157 S158 S159 S160 S161 S162 L41 L42 L43 L44 L45 L46 S163 S164 S165 S166 S167 S168 S169 bodies 1
move_face "MoveFace1" to x (1, 0, 0) y (0, 0.996195, -0.087156) z (0, 0.087156, 0.996195) at (0, 0.0475, -8.6295) 6 faces at (-162.9162, -98.8, -4.8556) (-132.1162, -98.8, -4.8556) (-101.3162, -98.8, -4.8556) (-70.5162, -98.8, -4.8556) (-40.6564, -98.8, -5.801) (-9.8564, -98.8, -5.801) on bodies 1
sketch "Sketch9" plane through (3, 0, 0) normal (1, 0, 0) x (0, 1, 0)
  line L0 (0, -10) -> (-26.1075, 45)
  line L1 (-26.1075, 45) -> (-76.4751, 45)
  line L2 (-76.4751, 45) -> (-91.0004, 7.1605)
  line L3 (-91.0004, 7.1605) -> (-95.4512, 8.869)
  line L4 (-95.4512, 8.869) -> (-99.3358, -1.2506)
  arc A0 (-99.3358, -1.2506) -> (-100.1992, -5.9094) centre (-87.1992, -5.9094) ccw
  line L5 (-100.1992, -5.9094) -> (-100.1992, -13.5)
  line L6 (-100.1992, -13.5) -> (0, -13.5)
  line L7 (0, -13.5) -> (0, -10)
  line L8 (-76.4751, 45) -> (-75.4, 47.8007)
  line L9 (-26.1075, 45) -> (-27.437, 47.8007)
  line L10 (-75.4, 47.8007) -> (-27.437, 47.8007)
  line L11 (-27.437, 47.8007) -> (-24.437, 47.8007)
  line L12 (-24.437, 47.8007) -> (4.6614, -13.5)
  line L13 (4.6614, -13.5) -> (0, -13.5)
  line L14 (0, -10) -> (0, -13.5)
  line L15 (0, -10) -> (-26.1075, 45)
  line L16 (-26.1075, 45) -> (-76.4751, 45)
  dimension "d39" = 3
  dimension "d41" = 3
  constraint coincident L1.end L2.start
  constraint parallel L2 L8
  constraint coincident L0.end L1.start
  constraint parallel L0 L9
  constraint parallel L10 L11
  constraint parallel L9 L12
  constraint coincident L6.end L7.start
  constraint perpendicular L7 L13
  constraint coincident L0.start L7.end
  constraint parallel L10 L16
  measures "d39" distance of L1.end L8.end
  measures "d41" distance of L9.end L11.end
extrude "Extrude10" add sketch "Sketch9" against normal blind 180 separate body contours L1 L8 L9 L10 L16 makes body 2
extrude "Extrude11" add sketch "Sketch9" against normal blind 180 separate body contours L0 L7 L9 L11 L12 L13 L14 L15 makes body 3
sketch "Sketch11" plane through (0, 0, 0) normal (-1, 0, 0) x (0, -1, 0)
  line L0 (26.1075, 45) -> (0, -10)
  line L1 (0, -10) -> (90, -10)
  line L2 (90, -10) -> (90, 0)
  line L3 (90, 0) -> (72.7261, 45)
  line L4 (72.7261, 45) -> (26.1075, 45)
  line L5 (74.6382, 40) -> (72.7261, 45)
  line L6 (74.6382, 40) -> (61, 40)
  line L7 (61, 40) -> (57.9944, 44.9835)
  line L8 (57.9944, 44.9835) -> (72.7261, 45)
  constraint coincident L3.end L4.start
  constraint parallel L4 L6
extrude "Extrude12" add sketch "Sketch11" along normal blind 10 contours L5 L6 L7 L8 bodies 2
extrude "Extrude13" add 1 faces at (-10, -63.9068, 43.3278) along direction (1, 0, 0) blind 10 from surface at -164 on bodies 2 bodies 2
sketch "Sketch12" plane through (0, 0, 47.8007) normal (0, 0, 1) x (-1, 0, 0)
  line L0 (-3, 75.4) -> (-3, 27.437)
  line L1 (-3, 27.437) -> (177, 27.437)
  line L2 (177, 27.437) -> (177, 75.4)
  line L3 (177, 75.4) -> (-3, 75.4)
  line L4 (-3, 75.4) -> (177, 75.4) construction
  line L5 (87, 75.4) -> (87, 27.437) construction
  line L6 (-3, 51.4185) -> (177, 51.4185) construction
  line L7 (93, 43.4185) -> (81, 43.4185)
  line L8 (81, 43.4185) -> (81, 59.4185)
  line L9 (81, 59.4185) -> (93, 59.4185)
  line L10 (93, 59.4185) -> (93, 43.4185)
  line L11 (93, 43.4185) -> (81, 59.4185) construction
  line L12 (81, 43.4185) -> (93, 59.4185) construction
  line L13 (38, 59.4185) -> (38, 43.4185)
  line L14 (26, 59.4185) -> (38, 59.4185)
  line L15 (26, 43.4185) -> (26, 59.4185)
  line L16 (38, 43.4185) -> (26, 43.4185)
  line L17 (148, 59.4185) -> (148, 43.4185)
  line L18 (136, 59.4185) -> (148, 59.4185)
  line L19 (136, 43.4185) -> (136, 59.4185)
  line L20 (148, 43.4185) -> (136, 43.4185)
  line L21 (32, 59.4185) -> (32, 43.4185) construction
  line L22 (142, 59.4185) -> (142, 43.4185) construction
  circle A0 centre (32, 51.4185) radius 3.513
  circle A1 centre (32, 51.4185) radius 4.513
  line L23 (145.8877, 48.2348) -> (145.1802, 47.528)
  line L24 (145.1802, 47.528) -> (138.1123, 54.6022)
  line L25 (138.1123, 54.6022) -> (138.8198, 55.309)
  line L26 (138.8198, 55.309) -> (145.8877, 48.2348)
  line L27 (145.8877, 48.2348) -> (138.1123, 54.6022) construction
  line L28 (145.1802, 47.528) -> (138.8198, 55.309) construction
  line L29 (145.8891, 54.669) -> (138.818, 47.5979)
  line L30 (145.182, 55.3761) -> (145.8891, 54.669)
  line L31 (138.1109, 48.305) -> (145.182, 55.3761)
  line L32 (138.818, 47.5979) -> (138.1109, 48.305)
  line L33 (83, 52) -> (91, 52)
  line L34 (91, 52) -> (91, 51)
  line L35 (91, 51) -> (83, 51)
  line L36 (83, 51) -> (83, 52)
  circle A2 centre (32, 51.4185) radius 7.5
  circle A3 centre (87, 51.4185) radius 7.5
  circle A4 centre (142, 51.4185) radius 7.5
  point P0 (87, 51.4185)
  point P1 (142, 51.4185)
  dimension "d51" = 12
  dimension "d52" = 16
  dimension "d55" = 55
  dimension "d56" = 0
  dimension "d57" = 1
  dimension "d58" = 10
  dimension "d59" = 1
  dimension "d60" = 10
  dimension "d61" = 15
  dimension "d62" = 15
  dimension "d63" = 15
  constraint coincident L0.start L3.end
  constraint coincident L2.end L3.start
  constraint midpoint L3 L5.start
  constraint midpoint L1 L5.end
  constraint midpoint L0 L6.start
  constraint midpoint L2 L6.end
  constraint horizontal L7
  constraint perpendicular L7 L8
  constraint parallel L7 L9
  constraint parallel L8 L10
  constraint coincident L11 P0
  constraint coincident L12 P0
  constraint midpoint L6 P0
  constraint midpoint L14 L21.start
  constraint midpoint L16 L21.end
  constraint midpoint L18 L22.start
  constraint midpoint L20 L22.end
  constraint midpoint L21 A0.centre
  constraint concentric A0 A1
  constraint perpendicular L23 L24
  constraint parallel L23 L25
  constraint parallel L24 L26
  constraint coincident L27 P1
  constraint coincident L28 P1
  constraint midpoint L22 P1
  constraint perpendicular L31 L32
  constraint parallel L30 L32
  constraint parallel L29 L31
  constraint horizontal L33
  constraint vertical L34
  constraint horizontal L35
  constraint vertical L36
  constraint concentric A1 A2
  constraint coincident P0 A3.centre
  constraint coincident P1 A4.centre
  measures "d51" distance of L8.end L9.end
  measures "d52" distance of L7.end L8.end
  measures "d57" distance of L24.end L25.end
  measures "d58" distance of L23.end L24.end
  measures "d59" distance of L29.start L30.start
  measures "d60" distance of L31.start L30.start
  measures "d61" diameter of A2
  measures "d62" diameter of A3
  measures "d63" diameter of A4
extrude "Extrude14" cut sketch "Sketch12" against normal blind 1 contours L8 L10 A3 | L10 A3 | L8 A3 | L13 A2 | L13 L15 A2 | L15 A2 | L17 A4 | L17 L19 A4 | L19 A4 | A0 | A1 | L23 L24 L26 L29 | L24 L26 L29 L31 | L26 L29 L30 L31 | L24 L29 L31 L32 | L24 L25 L26 L31 | L33 L34 L35 L36 bodies 2
extrude "Extrude15" [suppressed]
fillet "Fillet2" radius 5 3 edges at (-135.0075, -54.1306, 46.8007) (-80.0075, -54.1306, 46.8007) (-25.0075, -54.1306, 46.8007) on bodies 2
extrude "Extrude16" add sketch "Sketch12" against normal blind 1 from surface at -2.8007 contours L7 L8 L10 A3 | L8 L10 A3 | L8 L9 L10 A3 | L13 L14 L15 A2 | L13 L15 A2 | L13 L15 L16 A2 | L17 L18 L19 A4 | L17 L19 A4 | L17 L19 L20 A4 | A0 | A1 | L23 L24 L26 L29 | L24 L26 L29 L31 | L26 L29 L30 L31 | L24 L29 L31 L32 | L24 L25 L26 L31 | L33 L34 L35 L36 bodies 2
move_face "OffsetFaces1" offset -5 3 faces at (-34, -43.4185, 44.6667) (-89, -43.4185, 44.6667) (-144, -43.4185, 44.6667) on bodies 2
fillet "Fillet3" radius 5 3 edges at (-80.0075, -54.1306, 47.8007) (-25.0075, -54.1306, 47.8007) (-135.0075, -54.1306, 47.8007) on bodies 2
sketch "Sketch13" plane through (0, -1.4256, -0.6767) normal (0, 0.903389, 0.428822) x (-1, 0, 0)
  line L0 (-3, 53.6618) -> (-3, -14.1947)
  line L1 (-3, -14.1947) -> (177, -14.1947)
  line L2 (177, -14.1947) -> (177, 53.6618)
  line L3 (177, 53.6618) -> (-3, 53.6618)
  line L4 (177, -14.1947) -> (169, -14.1947) construction
  line L5 (177, -14.1947) -> (156, -14.1947) construction
  line L6 (156, -14.1947) -> (169, -14.1947)
  line L7 (169, -14.1947) -> (169, 25.8053)
  line L8 (169, 25.8053) -> (156, 25.8053)
  line L9 (156, 25.8053) -> (156, -14.1947)
  line L10 (25, 44) -> (21.5359, 42)
  line L11 (21.5359, 42) -> (21.5359, 38)
  line L12 (21.5359, 38) -> (25, 36)
  line L13 (25, 36) -> (28.4641, 38)
  line L14 (28.4641, 38) -> (28.4641, 42)
  line L15 (28.4641, 42) -> (25, 44)
  line L16 (28.5, 28) -> (31.9641, 30)
  line L17 (25.0359, 30) -> (28.5, 28)
  line L18 (31.9641, 34) -> (28.5, 36)
  line L19 (28.5, 36) -> (25.0359, 34)
  line L20 (31.9641, 30) -> (31.9641, 34)
  line L21 (25.0359, 34) -> (25.0359, 30)
  line L22 (34, 44) -> (30.5359, 42)
  line L23 (34.0359, 34) -> (34.0359, 30)
  line L24 (37.4641, 42) -> (34, 44)
  line L25 (30.5359, 42) -> (30.5359, 38)
  line L26 (40.9641, 30) -> (40.9641, 34)
  line L27 (37.5, 28) -> (40.9641, 30)
  line L28 (37.5, 36) -> (34.0359, 34)
  line L29 (30.5359, 38) -> (34, 36)
  line L30 (34.0359, 30) -> (37.5, 28)
  line L31 (40.9641, 34) -> (37.5, 36)
  line L32 (37.4641, 38) -> (37.4641, 42)
  line L33 (34, 36) -> (37.4641, 38)
  line L34 (43, 44) -> (39.5359, 42)
  line L35 (43.0359, 34) -> (43.0359, 30)
  line L36 (46.4641, 42) -> (43, 44)
  line L37 (39.5359, 42) -> (39.5359, 38)
  line L38 (49.9641, 30) -> (49.9641, 34)
  line L39 (46.5, 28) -> (49.9641, 30)
  line L40 (46.5, 36) -> (43.0359, 34)
  line L41 (39.5359, 38) -> (43, 36)
  line L42 (43.0359, 30) -> (46.5, 28)
  line L43 (49.9641, 34) -> (46.5, 36)
  line L44 (46.4641, 38) -> (46.4641, 42)
  line L45 (43, 36) -> (46.4641, 38)
  line L46 (52, 44) -> (48.5359, 42)
  line L47 (52.0359, 34) -> (52.0359, 30)
  line L48 (55.4641, 42) -> (52, 44)
  line L49 (48.5359, 42) -> (48.5359, 38)
  line L50 (58.9641, 30) -> (58.9641, 34)
  line L51 (55.5, 28) -> (58.9641, 30)
  line L52 (55.5, 36) -> (52.0359, 34)
  line L53 (48.5359, 38) -> (52, 36)
  line L54 (52.0359, 30) -> (55.5, 28)
  line L55 (58.9641, 34) -> (55.5, 36)
  line L56 (55.4641, 38) -> (55.4641, 42)
  line L57 (52, 36) -> (55.4641, 38)
  line L58 (61, 44) -> (57.5359, 42)
  line L59 (61.0359, 34) -> (61.0359, 30)
  line L60 (64.4641, 42) -> (61, 44)
  line L61 (57.5359, 42) -> (57.5359, 38)
  line L62 (67.9641, 30) -> (67.9641, 34)
  line L63 (64.5, 28) -> (67.9641, 30)
  line L64 (64.5, 36) -> (61.0359, 34)
  line L65 (57.5359, 38) -> (61, 36)
  line L66 (61.0359, 30) -> (64.5, 28)
  line L67 (67.9641, 34) -> (64.5, 36)
  line L68 (64.4641, 38) -> (64.4641, 42)
  line L69 (61, 36) -> (64.4641, 38)
  line L70 (70, 44) -> (66.5359, 42)
  line L71 (70.0359, 34) -> (70.0359, 30)
  line L72 (73.4641, 42) -> (70, 44)
  line L73 (66.5359, 42) -> (66.5359, 38)
  line L74 (76.9641, 30) -> (76.9641, 34)
  line L75 (73.5, 28) -> (76.9641, 30)
  line L76 (73.5, 36) -> (70.0359, 34)
  line L77 (66.5359, 38) -> (70, 36)
  line L78 (70.0359, 30) -> (73.5, 28)
  line L79 (76.9641, 34) -> (73.5, 36)
  line L80 (73.4641, 38) -> (73.4641, 42)
  line L81 (70, 36) -> (73.4641, 38)
  line L82 (25, 28) -> (21.5359, 26)
  line L83 (25.0359, 18) -> (25.0359, 14)
  line L84 (28.4641, 26) -> (25, 28)
  line L85 (21.5359, 26) -> (21.5359, 22)
  line L86 (31.9641, 14) -> (31.9641, 18)
  line L87 (28.5, 12) -> (31.9641, 14)
  line L88 (28.5, 20) -> (25.0359, 18)
  line L89 (21.5359, 22) -> (25, 20)
  line L90 (25.0359, 14) -> (28.5, 12)
  line L91 (31.9641, 18) -> (28.5, 20)
  line L92 (28.4641, 22) -> (28.4641, 26)
  line L93 (25, 20) -> (28.4641, 22)
  line L94 (34, 28) -> (30.5359, 26)
  line L95 (34.0359, 18) -> (34.0359, 14)
  line L96 (37.4641, 26) -> (34, 28)
  line L97 (30.5359, 26) -> (30.5359, 22)
  line L98 (40.9641, 14) -> (40.9641, 18)
  line L99 (37.5, 12) -> (40.9641, 14)
  line L100 (37.5, 20) -> (34.0359, 18)
  line L101 (30.5359, 22) -> (34, 20)
  line L102 (34.0359, 14) -> (37.5, 12)
  line L103 (40.9641, 18) -> (37.5, 20)
  line L104 (37.4641, 22) -> (37.4641, 26)
  line L105 (34, 20) -> (37.4641, 22)
  line L106 (43, 28) -> (39.5359, 26)
  line L107 (43.0359, 18) -> (43.0359, 14)
  line L108 (46.4641, 26) -> (43, 28)
  line L109 (39.5359, 26) -> (39.5359, 22)
  line L110 (49.9641, 14) -> (49.9641, 18)
  line L111 (46.5, 12) -> (49.9641, 14)
  line L112 (46.5, 20) -> (43.0359, 18)
  line L113 (39.5359, 22) -> (43, 20)
  line L114 (43.0359, 14) -> (46.5, 12)
  line L115 (49.9641, 18) -> (46.5, 20)
  line L116 (46.4641, 22) -> (46.4641, 26)
  line L117 (43, 20) -> (46.4641, 22)
  line L118 (52, 28) -> (48.5359, 26)
  line L119 (52.0359, 18) -> (52.0359, 14)
  line L120 (55.4641, 26) -> (52, 28)
  line L121 (48.5359, 26) -> (48.5359, 22)
  line L122 (58.9641, 14) -> (58.9641, 18)
  line L123 (55.5, 12) -> (58.9641, 14)
  line L124 (55.5, 20) -> (52.0359, 18)
  line L125 (48.5359, 22) -> (52, 20)
  line L126 (52.0359, 14) -> (55.5, 12)
  line L127 (58.9641, 18) -> (55.5, 20)
  line L128 (55.4641, 22) -> (55.4641, 26)
  line L129 (52, 20) -> (55.4641, 22)
  line L130 (61, 28) -> (57.5359, 26)
  line L131 (61.0359, 18) -> (61.0359, 14)
  line L132 (64.4641, 26) -> (61, 28)
  line L133 (57.5359, 26) -> (57.5359, 22)
  line L134 (67.9641, 14) -> (67.9641, 18)
  line L135 (64.5, 12) -> (67.9641, 14)
  line L136 (64.5, 20) -> (61.0359, 18)
  line L137 (57.5359, 22) -> (61, 20)
  line L138 (61.0359, 14) -> (64.5, 12)
  line L139 (67.9641, 18) -> (64.5, 20)
  line L140 (64.4641, 22) -> (64.4641, 26)
  line L141 (61, 20) -> (64.4641, 22)
  line L142 (70, 28) -> (66.5359, 26)
  line L143 (70.0359, 18) -> (70.0359, 14)
  line L144 (73.4641, 26) -> (70, 28)
  line L145 (66.5359, 26) -> (66.5359, 22)
  line L146 (76.9641, 14) -> (76.9641, 18)
  line L147 (73.5, 12) -> (76.9641, 14)
  line L148 (73.5, 20) -> (70.0359, 18)
  line L149 (66.5359, 22) -> (70, 20)
  line L150 (70.0359, 14) -> (73.5, 12)
  line L151 (76.9641, 18) -> (73.5, 20)
  line L152 (73.4641, 22) -> (73.4641, 26)
  line L153 (70, 20) -> (73.4641, 22)
  line L154 (25, 12) -> (21.5359, 10)
  line L155 (25.0359, 2) -> (25.0359, -2)
  line L156 (28.4641, 10) -> (25, 12)
  line L157 (21.5359, 10) -> (21.5359, 6)
  line L158 (31.9641, -2) -> (31.9641, 2)
  line L159 (28.5, -4) -> (31.9641, -2)
  line L160 (28.5, 4) -> (25.0359, 2)
  line L161 (21.5359, 6) -> (25, 4)
  line L162 (25.0359, -2) -> (28.5, -4)
  line L163 (31.9641, 2) -> (28.5, 4)
  line L164 (28.4641, 6) -> (28.4641, 10)
  line L165 (25, 4) -> (28.4641, 6)
  line L166 (34, 12) -> (30.5359, 10)
  line L167 (34.0359, 2) -> (34.0359, -2)
  line L168 (37.4641, 10) -> (34, 12)
  line L169 (30.5359, 10) -> (30.5359, 6)
  line L170 (40.9641, -2) -> (40.9641, 2)
  line L171 (37.5, -4) -> (40.9641, -2)
  line L172 (37.5, 4) -> (34.0359, 2)
  line L173 (30.5359, 6) -> (34, 4)
  line L174 (34.0359, -2) -> (37.5, -4)
  line L175 (40.9641, 2) -> (37.5, 4)
  line L176 (37.4641, 6) -> (37.4641, 10)
  line L177 (34, 4) -> (37.4641, 6)
  line L178 (43, 12) -> (39.5359, 10)
  line L179 (43.0359, 2) -> (43.0359, -2)
  line L180 (46.4641, 10) -> (43, 12)
  line L181 (39.5359, 10) -> (39.5359, 6)
  line L182 (49.9641, -2) -> (49.9641, 2)
  line L183 (46.5, -4) -> (49.9641, -2)
  line L184 (46.5, 4) -> (43.0359, 2)
  line L185 (39.5359, 6) -> (43, 4)
  line L186 (43.0359, -2) -> (46.5, -4)
  line L187 (49.9641, 2) -> (46.5, 4)
  line L188 (46.4641, 6) -> (46.4641, 10)
  line L189 (43, 4) -> (46.4641, 6)
  line L190 (52, 12) -> (48.5359, 10)
  line L191 (52.0359, 2) -> (52.0359, -2)
  line L192 (55.4641, 10) -> (52, 12)
  line L193 (48.5359, 10) -> (48.5359, 6)
  line L194 (58.9641, -2) -> (58.9641, 2)
  line L195 (55.5, -4) -> (58.9641, -2)
  line L196 (55.5, 4) -> (52.0359, 2)
  line L197 (48.5359, 6) -> (52, 4)
  line L198 (52.0359, -2) -> (55.5, -4)
  line L199 (58.9641, 2) -> (55.5, 4)
  line L200 (55.4641, 6) -> (55.4641, 10)
  line L201 (52, 4) -> (55.4641, 6)
  line L202 (61, 12) -> (57.5359, 10)
  line L203 (61.0359, 2) -> (61.0359, -2)
  line L204 (64.4641, 10) -> (61, 12)
  line L205 (57.5359, 10) -> (57.5359, 6)
  line L206 (67.9641, -2) -> (67.9641, 2)
  line L207 (64.5, -4) -> (67.9641, -2)
  line L208 (64.5, 4) -> (61.0359, 2)
  line L209 (57.5359, 6) -> (61, 4)
  line L210 (61.0359, -2) -> (64.5, -4)
  line L211 (67.9641, 2) -> (64.5, 4)
  line L212 (64.4641, 6) -> (64.4641, 10)
  line L213 (61, 4) -> (64.4641, 6)
  line L214 (70, 12) -> (66.5359, 10)
  line L215 (70.0359, 2) -> (70.0359, -2)
  line L216 (73.4641, 10) -> (70, 12)
  line L217 (66.5359, 10) -> (66.5359, 6)
  line L218 (76.9641, -2) -> (76.9641, 2)
  line L219 (73.5, -4) -> (76.9641, -2)
  line L220 (73.5, 4) -> (70.0359, 2)
  line L221 (66.5359, 6) -> (70, 4)
  line L222 (70.0359, -2) -> (73.5, -4)
  line L223 (76.9641, 2) -> (73.5, 4)
  line L224 (73.4641, 6) -> (73.4641, 10)
  line L225 (70, 4) -> (73.4641, 6)
  point P0 (25, 40)
  point P1 (28.5, 32)
  point P2 (34, 40)
  point P3 (37.5, 32)
  point P4 (43, 40)
  point P5 (46.5, 32)
  point P6 (52, 40)
  point P7 (55.5, 32)
  point P8 (61, 40)
  point P9 (64.5, 32)
  point P10 (70, 40)
  point P11 (73.5, 32)
  point P12 (25, 24)
  point P13 (28.5, 16)
  point P14 (34, 24)
  point P15 (37.5, 16)
  point P16 (43, 24)
  point P17 (46.5, 16)
  point P18 (52, 24)
  point P19 (55.5, 16)
  point P20 (61, 24)
  point P21 (64.5, 16)
  point P22 (70, 24)
  point P23 (73.5, 16)
  point P24 (25, 8)
  point P25 (28.5, 0)
  point P26 (34, 8)
  point P27 (37.5, 0)
  point P28 (43, 8)
  point P29 (46.5, 0)
  point P30 (52, 8)
  point P31 (55.5, 0)
  point P32 (61, 8)
  point P33 (64.5, 0)
  point P34 (70, 8)
  point P35 (73.5, 0)
  dimension "d76" = 8
  dimension "d77" = 21
  dimension "d78" = 40
  dimension "d81" = 45
  dimension "d82" = -32
  constraint coincident L1.end L2.start
  constraint perpendicular L2 L4
  constraint perpendicular L2 L5
  constraint horizontal L6
  constraint vertical L7
  constraint horizontal L8
  constraint vertical L9
  measures "d76" distance of L1.end L4.end
  measures "d77" distance of L1.end L5.end
  measures "d78" distance of L5.end L8.end
extrude "Extrude17" cut sketch "Sketch13" against normal blind 15 contours L10 L11 L12 L13 L14 L15 | L16 L17 L18 L19 L20 L21 | L22 L24 L25 L29 L32 L33 | L23 L26 L27 L28 L30 L31 | L34 L36 L37 L41 L44 L45 | L35 L38 L39 L40 L42 L43 | L46 L48 L49 L53 L56 L57 | L47 L50 L51 L52 L54 L55 | L58 L60 L61 L65 L68 L69 | L59 L62 L63 L64 L66 L67 | L70 L72 L73 L77 L80 L81 | L71 L74 L75 L76 L78 L79 | L82 L84 L85 L89 L92 L93 | L83 L86 L87 L88 L90 L91 | L94 L96 L97 L101 L104 L105 | L95 L98 L99 L100 L102 L103 | L106 L108 L109 L113 L116 L117 | L107 L110 L111 L112 L114 L115 | L118 L120 L121 L125 L128 L129 | L119 L122 L123 L124 L126 L127 | L130 L132 L133 L137 L140 L141 | L131 L134 L135 L136 L138 L139 | L142 L144 L145 L149 L152 L153 | L143 L146 L147 L148 L150 L151 | L154 L156 L157 L161 L164 L165 | L155 L158 L159 L160 L162 L163 | L166 L168 L169 L173 L176 L177 | L167 L170 L171 L172 L174 L175 | L178 L180 L181 L185 L188 L189 | L179 L182 L183 L184 L186 L187 | L190 L192 L193 L197 L200 L201 | L191 L194 L195 L196 L198 L199 | L202 L204 L205 L209 L212 L213 | L203 L206 L207 L208 L210 L211 | L214 L216 L217 L221 L224 L225 | L215 L218 L219 L220 L222 L223 bodies 3
extrude "Extrude18" cut sketch "Sketch13" against normal blind 20 contours L1 L6 L7 L8 L9 bodies 3
equation "d22 = ( 4 / 2 ) * 1 mm"
